Autodesk Inventor part; units mm, degrees
(part 2 of 2)
sketch "Эскиз17" plane through (0, 13, 0) normal (0, 1, 0) x (1, 0, 0)
  arc A0 (13, -62.9053) -> (8.25, -61.7214) centre (0, -104.941) ccw projected
  line L0 (11.5, -48.5381) -> (11.5, -67.0381) projected
  line L1 (8.25, -36.2214) -> (8.25, -61.7214) projected
  line L2 (11.5, -48.5381) -> (13, -48.5381) projected
  line L3 (11.5, -48.5381) -> (8.25, -48.5381)
  line L4 (0, -67.941) -> (0, -60.941) construction
  line L5 (-11.5, -48.5381) -> (-8.25, -48.5381)
  arc A1 (-8.25, -61.7214) -> (-13, -62.9053) centre (0, -104.941) ccw projected
  line L6 (-8.25, -36.2214) -> (-8.25, -61.7214) projected
  line L7 (-11.5, -48.5381) -> (-11.5, -67.0381) projected
  line L8 (13, -48.5381) -> (13, -62.9053) projected
  line L9 (15, -48.5381) -> (13, -48.5381) projected
  line L10 (15, -63.3086) -> (15, -48.5381) projected
  line L11 (14.893, -63.5381) -> (15, -63.3086) projected
  arc A2 (14.893, -63.5381) -> (13, -62.9053) centre (0, -104.941) ccw projected
  line L12 (-13, -62.9053) -> (-13, -48.5381) projected
  arc A3 (-13, -62.9053) -> (-14.893, -63.5381) centre (0, -104.941) ccw projected
  line L13 (-15, -63.3086) -> (-14.893, -63.5381) projected
  line L14 (-15, -48.5381) -> (-15, -63.3086) projected
  line L15 (-13, -48.5381) -> (-15, -48.5381) projected
  line L16 (-13, -48.5381) -> (-11.5, -48.5381) projected
  line L17 (-11.5, -48.5381) -> (-13, -48.5381)
  point P0 (0, 0)
  point P1 (-13, -62.9053)
  constraints: 6 end point, 3 symmetric about line, 1 collinear, 1 perpendicular, 1 point on line
extrude "Выдавливание16" add sketch "Эскиз17" along normal blind 4.5 contours A0 L0 L2 L8 | A0 L1 L3 L0 | L5 L6 A1 L7 | L7 A1 L12 L16
extrude "Выдавливание17" add sketch "Эскиз13" along normal blind 13
chamfer "Фаска1" distance 3 angle 45 1 edges at (4.5, 13, 40)
ref_plane "РабПлоскость4" through (14.893, 35, 48.5381) normal (0, -0.0000001, -1) x (-1, 0, 0)
sketch "Эскиз18" plane through (14.893, 35, 48.5381) normal (0, -0.0000001, -1) x (-1, 0, 0)
  line L0 (29.893, 0) -> (27.893, 0) construction
  line L1 (27.893, 0) -> (27.893, -4.5) construction
  line L2 (27.893, -4.5) -> (26.393, -6) projected
  line L3 (26.393, -6) -> (26.393, -9) projected
  line L4 (26.393, -9) -> (27.893, -9) projected
  line L5 (27.893, -9) -> (27.893, -15) construction
  line L6 (27.893, -15) -> (29.893, -15) construction
  line L7 (29.893, -15) -> (29.893, 0) construction
  line L8 (1.893, -4.5) -> (1.893, 0) construction
  line L9 (1.893, 0) -> (-0.107, 0) construction
  line L10 (-0.107, 0) -> (-0.107, -15) construction
  line L11 (-0.107, -15) -> (1.893, -15) construction
  line L12 (1.893, -15) -> (1.893, -9) construction
  line L13 (1.893, -9) -> (3.393, -9) projected
  line L14 (3.393, -9) -> (3.393, -6) projected
  line L15 (3.393, -6) -> (1.893, -4.5) projected
  line L16 (27.893, -4.5) -> (27.893, -9)
  line L17 (1.893, -4.5) -> (1.893, -9) projected
  line L18 (1.893, -9) -> (1.893, -4.5)
  line L19 (3.393, -9) -> (1.893, -9) projected
  line L20 (1.893, -9) -> (3.393, -7.5)
  line L21 (3.393, -6) -> (3.393, -9) projected
  line L22 (27.893, -9) -> (26.393, -7.5)
  line L23 (26.393, -6) -> (26.393, -9) projected
  point P0 (14.893, -35)
  point P1 (26.393, -7.5)
  point P2 (3.393, -7.5)
  constraints: 8 end point, 2 midpoint, 1 collinear, 1 vertical
extrude "Выдавливание18" cut sketch "Эскиз18" against normal blind 8 contours L16 L22 L3 L2 | L17 L15 L14 L20
extrude "Выдавливание19" cut sketch "Эскиз18" against normal blind 80 contours L4 L3 L22 | L20 L14 L13
sketch "Эскиз19" plane through (0, 35, 0) normal (0, 1, 0) x (1, 0, 0)
  line L0 (-15, -63.3086) -> (-16.9326, -59.1641) projected
  arc A0 (-16.9326, -59.1641) -> (-24.1831, -62.545) centre (-20.5578, -60.8546) ccw projected
  line L1 (-24.1831, -62.545) -> (-22.1434, -66.9191) projected
  arc A1 (-22.1434, -66.9191) -> (-28.5452, -71.4571) centre (0, -104.941) ccw projected
  line L2 (-28.5452, -71.4571) -> (-31.2232, -73.7044) projected
  arc A2 (-31.2232, -73.7044) -> (-26.8032, -79.1314) centre (-28.9734, -76.3855) ccw projected
  line L3 (-26.8032, -79.1314) -> (-23.7825, -76.5969) projected
  arc A3 (-13, -70.3) -> (-23.7825, -76.5969) centre (0, -104.941) ccw projected
  line L4 (-13, -70.3) -> (-13, -62.9053) projected
  arc A4 (-13, -62.9053) -> (-14.893, -63.5381) centre (0, -104.941) ccw projected
  line L5 (-14.893, -63.5381) -> (-15, -63.3086) projected
  circle A5 centre (-20.5578, -60.8546) radius 2 projected
  circle A6 centre (20.5578, -60.8546) radius 2 projected
  line L6 (15, -63.3086) -> (14.893, -63.5381) projected
  arc A7 (14.893, -63.5381) -> (13, -62.9053) centre (0, -104.941) ccw projected
  line L7 (13, -62.9053) -> (13, -70.3) projected
  arc A8 (23.7825, -76.5969) -> (13, -70.3) centre (0, -104.941) ccw projected
  line L8 (23.7825, -76.5969) -> (26.8032, -79.1314) projected
  arc A9 (26.8032, -79.1314) -> (31.2232, -73.7044) centre (28.9734, -76.3855) ccw projected
  line L9 (31.2232, -73.7044) -> (28.5452, -71.4571) projected
  arc A10 (28.5452, -71.4571) -> (22.1434, -66.9191) centre (0, -104.941) ccw projected
  line L10 (22.1434, -66.9191) -> (24.1831, -62.545) projected
  arc A11 (24.1831, -62.545) -> (16.9326, -59.1641) centre (20.5578, -60.8546) ccw projected
  line L11 (16.9326, -59.1641) -> (15, -63.3086) projected
  point P0 (0, 0)
extrude "Выдавливание20" add sketch "Эскиз19" along normal blind 4
sketch "Эскиз20" plane through (0, 0, 0) normal (0, -1, 0) x (1, 0, 0)
  line L0 (34.5044, 86.1738) -> (-28.4923, 86.1738)
  line L1 (-28.4923, 86.1738) -> (-28.4923, 22.393)
  line L2 (-28.4923, 22.393) -> (34.5044, 22.393)
  line L3 (34.5044, 22.393) -> (34.5044, 86.1738)
  point P0 (0, 0)
  constraints: 8 end point, 2 parallel, 1 horizontal, 1 perpendicular
extrude "Выдавливание21" cut sketch "Эскиз20" against normal blind 4
